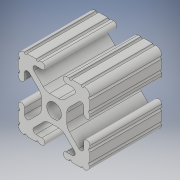
# Autodesk Inventor part: 1010-20''-CL
Saved by Autodesk Inventor 2018 (Build 220112000, 112)
## iProperties
Created: 2020-01-26
Part Number: 1010-20''-CL
Material: Generic
Document SubType Name: Modeling
Designer: s-4008082
Density: 1 g/cm^3
Appearance: Default
Author: s-4008082
Autodesk Inventor part; units mm, degrees
ref_plane "YZ Plane" through (0, 0, 0) normal (1, 0, 0) x (0, 1, 0)
ref_plane "XZ Plane" through (0, 0, 0) normal (0, 1, 0) x (-1, 0, 0)
ref_plane "XY Plane" through (0, 0, 0) normal (0, 0, 1) x (1, 0, 0)
sketch "Sketch1" plane through (0, 0, 0) normal (0, 0, 1) x (1, 0, 0)
  arc A0 (-12.6998, -10.5664) -> (-10.5664, -12.6998) centre (-10.5918, -10.5918) ccw
  arc A1 (-9.5504, -12.7) -> (-10.5664, -12.6998) centre (-10.0584, -12.7) ccw
  line L0 (-9.5504, -12.7) -> (-6.3331, -12.7)
  arc A2 (-5.3171, -12.7) -> (-6.3331, -12.7) centre (-5.8251, -12.7) ccw
  line L1 (-5.3171, -12.7) -> (-4.3434, -12.7)
  arc A3 (-4.3434, -12.7) -> (-4.3434, -10.4902) centre (-4.3434, -11.5951) ccw
  line L2 (-4.3434, -10.4902) -> (-6.4748, -10.4902)
  arc A4 (-7.1932, -8.7558) -> (-6.4748, -10.4902) centre (-6.4748, -9.4742) ccw
  line L3 (-7.1932, -8.7558) -> (-3.8632, -5.4257)
  arc A5 (-1.6181, -4.4958) -> (-3.8632, -5.4257) centre (-1.6181, -7.6708) ccw
  line L4 (-1.6181, -4.4958) -> (1.6181, -4.4958)
  arc A6 (3.8632, -5.4257) -> (1.6181, -4.4958) centre (1.6181, -7.6708) ccw
  line L5 (3.8632, -5.4257) -> (7.1932, -8.7558)
  arc A7 (6.4748, -10.4902) -> (7.1932, -8.7558) centre (6.4748, -9.4742) ccw
  line L6 (6.4748, -10.4902) -> (4.3434, -10.4902)
  arc A8 (4.3434, -10.4902) -> (4.3434, -12.7) centre (4.3434, -11.5951) ccw
  line L7 (4.3434, -12.7) -> (5.3171, -12.7)
  arc A9 (6.3331, -12.7) -> (5.3171, -12.7) centre (5.8251, -12.7) ccw
  line L8 (6.3331, -12.7) -> (9.5504, -12.7)
  arc A10 (10.5664, -12.6998) -> (9.5504, -12.7) centre (10.0584, -12.7) ccw
  arc A11 (10.5664, -12.6998) -> (12.6998, -10.5664) centre (10.5918, -10.5918) ccw
  arc A12 (12.7, -9.5504) -> (12.6998, -10.5664) centre (12.7, -10.0584) ccw
  line L9 (12.7, -9.5504) -> (12.7, -6.3331)
  arc A13 (12.7, -5.3171) -> (12.7, -6.3331) centre (12.7, -5.8251) ccw
  line L10 (12.7, -5.3171) -> (12.7, -4.3434)
  arc A14 (12.7, -4.3434) -> (10.4902, -4.3434) centre (11.5951, -4.3434) ccw
  line L11 (10.4902, -4.3434) -> (10.4902, -6.4748)
  arc A15 (8.7558, -7.1932) -> (10.4902, -6.4748) centre (9.4742, -6.4748) ccw
  line L12 (8.7558, -7.1932) -> (5.4257, -3.8632)
  arc A16 (4.4958, -1.6181) -> (5.4257, -3.8632) centre (7.6708, -1.6181) ccw
  line L13 (4.4958, -1.6181) -> (4.4958, 1.6181)
  arc A17 (5.4257, 3.8632) -> (4.4958, 1.6181) centre (7.6708, 1.6181) ccw
  line L14 (5.4257, 3.8632) -> (8.7558, 7.1932)
  arc A18 (10.4902, 6.4748) -> (8.7558, 7.1932) centre (9.4742, 6.4748) ccw
  line L15 (10.4902, 6.4748) -> (10.4902, 4.3434)
  arc A19 (10.4902, 4.3434) -> (12.7, 4.3434) centre (11.5951, 4.3434) ccw
  line L16 (12.7, 4.3434) -> (12.7, 5.3171)
  arc A20 (12.7, 6.3331) -> (12.7, 5.3171) centre (12.7, 5.8251) ccw
  line L17 (12.7, 6.3331) -> (12.7, 9.5504)
  arc A21 (12.6998, 10.5664) -> (12.7, 9.5504) centre (12.7, 10.0584) ccw
  arc A22 (12.6998, 10.5664) -> (10.5664, 12.6998) centre (10.5918, 10.5918) ccw
  arc A23 (9.5504, 12.7) -> (10.5664, 12.6998) centre (10.0584, 12.7) ccw
  line L18 (9.5504, 12.7) -> (6.3331, 12.7)
  arc A24 (5.3171, 12.7) -> (6.3331, 12.7) centre (5.8251, 12.7) ccw
  line L19 (5.3171, 12.7) -> (4.3434, 12.7)
  arc A25 (4.3434, 12.7) -> (4.3434, 10.4902) centre (4.3434, 11.5951) ccw
  line L20 (4.3434, 10.4902) -> (6.4748, 10.4902)
  arc A26 (7.1932, 8.7558) -> (6.4748, 10.4902) centre (6.4748, 9.4742) ccw
  line L21 (7.1932, 8.7558) -> (3.8632, 5.4257)
  arc A27 (1.6181, 4.4958) -> (3.8632, 5.4257) centre (1.6181, 7.6708) ccw
  line L22 (1.6181, 4.4958) -> (-1.6181, 4.4958)
  arc A28 (-3.8632, 5.4257) -> (-1.6181, 4.4958) centre (-1.6181, 7.6708) ccw
  line L23 (-3.8632, 5.4257) -> (-7.1932, 8.7558)
  arc A29 (-6.4748, 10.4902) -> (-7.1932, 8.7558) centre (-6.4748, 9.4742) ccw
  line L24 (-6.4748, 10.4902) -> (-4.3434, 10.4902)
  arc A30 (-4.3434, 10.4902) -> (-4.3434, 12.7) centre (-4.3434, 11.5951) ccw
  line L25 (-4.3434, 12.7) -> (-5.3171, 12.7)
  arc A31 (-6.3331, 12.7) -> (-5.3171, 12.7) centre (-5.8251, 12.7) ccw
  line L26 (-6.3331, 12.7) -> (-9.5504, 12.7)
  arc A32 (-10.5664, 12.6998) -> (-9.5504, 12.7) centre (-10.0584, 12.7) ccw
  arc A33 (-10.5664, 12.6998) -> (-12.6998, 10.5664) centre (-10.5918, 10.5918) ccw
  arc A34 (-12.7, 9.5504) -> (-12.6998, 10.5664) centre (-12.7, 10.0584) ccw
  line L27 (-12.7, 9.5504) -> (-12.7, 6.3331)
  arc A35 (-12.7, 5.3171) -> (-12.7, 6.3331) centre (-12.7, 5.8251) ccw
  line L28 (-12.7, 5.3171) -> (-12.7, 4.3434)
  arc A36 (-12.7, 4.3434) -> (-10.4902, 4.3434) centre (-11.5951, 4.3434) ccw
  line L29 (-10.4902, 4.3434) -> (-10.4902, 6.4748)
  arc A37 (-8.7558, 7.1932) -> (-10.4902, 6.4748) centre (-9.4742, 6.4748) ccw
  line L30 (-8.7558, 7.1932) -> (-5.4257, 3.8632)
  arc A38 (-4.4958, 1.6181) -> (-5.4257, 3.8632) centre (-7.6708, 1.6181) ccw
  line L31 (-4.4958, 1.6181) -> (-4.4958, -1.6181)
  arc A39 (-5.4257, -3.8632) -> (-4.4958, -1.6181) centre (-7.6708, -1.6181) ccw
  line L32 (-5.4257, -3.8632) -> (-8.7558, -7.1932)
  arc A40 (-10.4902, -6.4748) -> (-8.7558, -7.1932) centre (-9.4742, -6.4748) ccw
  line L33 (-10.4902, -6.4748) -> (-10.4902, -4.3434)
  arc A41 (-10.4902, -4.3434) -> (-12.7, -4.3434) centre (-11.5951, -4.3434) ccw
  line L34 (-12.7, -4.3434) -> (-12.7, -5.3171)
  arc A42 (-12.7, -6.3331) -> (-12.7, -5.3171) centre (-12.7, -5.8251) ccw
  line L35 (-12.7, -6.3331) -> (-12.7, -9.5504)
  arc A43 (-12.6998, -10.5664) -> (-12.7, -9.5504) centre (-12.7, -10.0584) ccw
  circle A44 centre (0, 0) radius 2.6035
  constraints: 88 point on circle, 72 end point, 45 centre point
extrude "Extrusion1" add sketch "Sketch1" along normal blind 25.4
body "Solid1"
